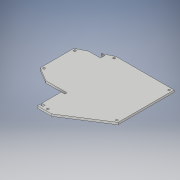
# Autodesk Inventor part: k2_l4
Saved by Autodesk Inventor 2017 (Build 210142000, 142)
## iProperties
Created: 2017-02-07
Part Number: k2_l4
Material: Generic
Document SubType Name: Modeling
Designer: herman
Density: 1 g/cm^3
Appearance: Default
Author: herman
Autodesk Inventor part; units mm, degrees
ref_plane "YZ Plane" through (0, 0, 0) normal (1, 0, 0) x (0, 1, 0)
ref_plane "XZ Plane" through (0, 0, 0) normal (0, 1, 0) x (-1, 0, 0)
ref_plane "XY Plane" through (0, 0, 0) normal (0, 0, 1) x (1, 0, 0)
sketch "Sketch8" plane through (0, 0, 0) normal (0, 1, 0) x (-1, 0, 0)
  line L0 (62.0619, 65.3949) -> (-60.9381, 65.3949) construction
  line L1 (-60.9381, 65.3949) -> (-60.9381, -51.6051) construction
  line L2 (-60.9381, -51.6051) -> (22.0619, -51.6051)
  line L3 (17.0619, 28.3949) -> (17.0619, 65.3949)
  line L4 (42.0619, 28.3949) -> (17.0619, 28.3949)
  line L5 (17.0619, 65.3949) -> (-2.9381, 65.3949)
  line L6 (-60.9381, 28.3949) -> (-60.9381, -51.6051)
  line L7 (-2.9381, 65.3949) -> (-60.9381, 28.3949)
  line L8 (42.0619, 28.3949) -> (62.0619, 16.3949)
  line L9 (62.0619, -31.6051) -> (22.0619, -51.6051)
  line L10 (62.0619, 16.3949) -> (62.0619, -31.6051)
  dimension "d120" = 123
  dimension "d122" = 20
  dimension "d123" = 80
  dimension "d124" = 117
  dimension "d125" = 123
  dimension "d128" = 37
  dimension "d129" = 40
  dimension "d131" = 20
  dimension "d147" = 12
  dimension "d154" = 20
  dimension "d155" = 25
  constraints: 22 end point, 3 point on line, 2 horizontal, 2 perpendicular, 1 collinear, 1 parallel, 1 vertical
  measures "d120" distance of L0.start L0.end
  measures "d122" distance of L3.end L5.end
  measures "d123" distance of L1.end L7.end
  measures "d124" vertical distance of L0.start L9.end
  measures "d125" distance from line of L1 L10.end
  measures "d128" distance of L3.end L3.start
  measures "d129" horizontal distance of L10.end L9.end
  measures "d131" vertical distance of L9.end L10.end
  measures "d147" vertical distance of L10.start L4.start
  measures "d154" horizontal distance of L10.start L4.start
  measures "d155" distance of L4.start L3.start
extrude "Extrusion9" add sketch "Sketch8" along normal blind 3
sketch "Sketch9" plane through (0, 3, 0) normal (0, 1, 0) x (1, 0, 0)
  line L0 (-17.0619, -28.3949) -> (-17.0619, -65.3949) construction
  line L1 (-17.0619, -65.3949) -> (2.9381, -65.3949) construction
  line L2 (2.9381, -65.3949) -> (60.9381, -28.3949) construction
  line L3 (60.9381, -28.3949) -> (60.9381, 51.6051) construction
  line L4 (60.9381, 51.6051) -> (-22.0619, 51.6051) construction
  line L5 (-22.0619, 51.6051) -> (-62.0619, 31.6051) construction
  line L6 (-62.0619, 31.6051) -> (-62.0619, -16.3949) construction
  line L7 (-62.0619, -16.3949) -> (-42.0619, -28.3949) construction
  line L8 (-42.0619, -28.3949) -> (-17.0619, -28.3949) construction
  line L9 (-13.5619, -61.8949) -> (-13.5619, -24.8949) construction
  line L10 (-13.5619, -24.8949) -> (-41.0924, -24.8949) construction
  line L11 (-41.0924, -24.8949) -> (-58.5619, -14.4133) construction
  line L12 (-58.5619, -14.4133) -> (-58.5619, 29.4419) construction
  line L13 (-58.5619, 29.4419) -> (-21.2357, 48.1051) construction
  line L14 (-21.2357, 48.1051) -> (57.4381, 48.1051) construction
  line L15 (57.4381, 48.1051) -> (57.4381, -26.4762) construction
  line L16 (57.4381, -26.4762) -> (1.9168, -61.8949) construction
  line L17 (1.9168, -61.8949) -> (-13.5619, -61.8949) construction
  circle A0 centre (-5.8226, -61.8949) radius 1.5
  circle A1 centre (57.4381, -26.4762) radius 1.5
  circle A2 centre (57.4381, 48.1051) radius 1.5
  circle A3 centre (-58.5619, 29.4419) radius 1.5
  circle A4 centre (-58.5619, -14.4133) radius 1.5
  circle A5 centre (-21.2357, 48.1051) radius 1.5
  point P0 (0, 0)
  dimension "d134" = 3.5
  dimension "d135" = 3
  dimension "d136" = 3
  dimension "d137" = 3
  dimension "d138" = 3
  dimension "d139" = 3
  dimension "d140" = 3
  constraints: 18 end point, 6 centre point, 5 coincident, 1 midpoint, 8 other
  measures "d134" distance between parallel lines of L0 L9
  measures "d135" diameter of A4
  measures "d136" diameter of A3
  measures "d137" diameter of A2
  measures "d138" diameter of A1
  measures "d139" diameter of A0
  measures "d140" diameter of A5
extrude "Extrusion10" cut sketch "Sketch9" against normal through all
sketch "Sketch10" plane through (0, 3, 0) normal (0, 1, 0) x (1, 0, 0)
  line L0 (-17.0619, -28.3949) -> (-17.0619, -65.3949) projected
  line L1 (-17.0619, -31.3949) -> (-12.0619, -31.3949)
  line L2 (-12.0619, -31.3949) -> (-12.0619, -28.3949)
  line L3 (-12.0619, -28.3949) -> (-17.0619, -28.3949)
  line L4 (-17.0619, -59.3949) -> (-12.0619, -59.3949)
  line L5 (-12.0619, -59.3949) -> (-12.0619, -62.3949)
  line L6 (-12.0619, -62.3949) -> (-17.0619, -62.3949)
  line L7 (-22.0619, 51.6051) -> (-62.0619, 31.6051) projected
  line L8 (-36.0619, 44.6051) -> (-31.0619, 44.6051)
  line L9 (-31.0619, 44.6051) -> (-31.0619, 38.6051)
  line L10 (-31.0619, 38.6051) -> (-48.0619, 38.6051)
  point P0 (0, 0)
  dimension "d143" = 3
  dimension "d144" = 3
  dimension "d145" = 5
  dimension "d146" = 28
  dimension "d148" = 6
  dimension "d149" = 5
  dimension "d150" = 7
  constraints: 18 end point, 7 point on line, 6 perpendicular, 1 horizontal, 1 parallel
  measures "d143" distance of L1.end L2.end
  measures "d144" distance of L4.end L5.end
  measures "d145" distance of L5.end L6.end
  measures "d146" distance of L1.start L4.start
  measures "d148" distance of L8.end L9.end
  measures "d149" distance of L8.start L8.end
  measures "d150" vertical distance of L8.end L7.start
extrude "Extrusion11" cut sketch "Sketch10" against normal through all
body "Solid5"
